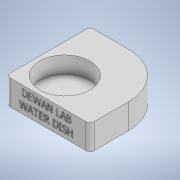
# Autodesk Inventor part: water dish holder_flat
Saved by Autodesk Inventor 2022.2 (Build 262287000, 287)
## iProperties
Created: 2022-03-09
Part Number: water dish holder_flat
Material: Generic
Document SubType Name: Modeling
Designer: dewanlab
Density: 1 g/cm^3
Appearance: Default
Author: dewanlab
Autodesk Inventor part; units mm, degrees
ref_plane "YZ Plane" through (0, 0, 0) normal (1, 0, 0) x (0, 1, 0)
ref_plane "XZ Plane" through (0, 0, 0) normal (0, 1, 0) x (-1, 0, 0)
ref_plane "XY Plane" through (0, 0, 0) normal (0, 0, 1) x (1, 0, 0)
sketch "Sketch1" plane through (0, 0, 0) normal (0, 1, 0) x (-1, 0, 0)
  line L0 (-31.75, -31.75) -> (31.75, -31.75)
  line L1 (31.75, -31.75) -> (31.75, 31.75)
  line L2 (31.75, 31.75) -> (-31.75, 31.75)
  line L3 (-31.75, 31.75) -> (-31.75, -31.75)
  line L4 (-31.75, -31.75) -> (31.75, 31.75) construction
  line L5 (31.75, -31.75) -> (-31.75, 31.75) construction
  point P0 (0, 0)
  dimension "d0" = 63.5
  dimension "d1" = 63.5
  constraints: 12 end point, 2 midpoint, 2 parallel, 1 horizontal, 1 perpendicular
  measures "d0" distance between parallel lines of L0 L2
  measures "d1" distance between parallel lines of L3 L1
extrude "Extrusion1" add sketch "Sketch1" along normal blind 19.05
fillet "Fillet1" radius 34.29 1 edges at (31.75, 9.525, -31.75)
sketch "Sketch2" plane through (0, 19.05, 0) normal (0, 1, 0) x (1, 0, 0)
  circle A0 centre (-9.525, -9.525) radius 19.05
  line L0 (-31.75, 31.75) -> (-31.75, -31.75) projected
  line L1 (-31.75, -31.75) -> (31.75, -31.75) projected
  point P0 (0, 0)
  dimension "d5" = 38.1
  dimension "d6" = 22.225
  dimension "d7" = 22.225
  constraints: 1 centre point
  measures "d5" diameter of A0
  measures "d6" distance from line of A0.centre L0
  measures "d7" distance from line of A0.centre L1
extrude "Extrusion2" cut sketch "Sketch2" against normal blind 12.7
fillet "Fillet2" radius 3.175 3 edges at (31.75, 9.525, 31.75) (-31.75, 9.525, 31.75) (-31.75, 9.525, -31.75)
sketch "Sketch4" plane through (-28.575, 0, 31.75) normal (0, 0, 1) x (1, 0, 0)
  line L0 (0.3237, 17.4668) -> (54.4444, 17.4668) construction
  line L1 (54.4444, 17.4668) -> (54.4444, 2.6465) construction
  line L2 (54.4444, 2.6465) -> (0.3237, 2.6465) construction
  line L3 (0.3237, 2.6465) -> (0.3237, 17.4668) construction
  spline S0 degree 2 poles (13.0168, 14.2799) (13.0168, 13.5841) (12.4528, 12.4644) (11.9794, 12.1515) knots 0 0 0 1 2 2 2
  spline S1 degree 2 poles (11.9794, 12.1515) (11.5924, 11.9087) (10.7979, 11.744) (10.1804, 11.744) knots 0 0 0 1 2 2 2
  line L4 (10.1804, 11.744) -> (9.0113, 11.744)
  line L5 (9.0113, 11.744) -> (9.0113, 16.824)
  line L6 (9.0113, 16.824) -> (10.1681, 16.824)
  spline S2 degree 2 poles (10.1681, 16.824) (10.8844, 16.824) (11.6995, 16.6099) (11.9876, 16.4205) knots 0 0 0 1 2 2 2
  spline S3 degree 2 poles (11.9876, 16.4205) (12.4775, 16.0953) (13.0168, 15.0209) (13.0168, 14.2799) knots 0 0 0 1 2 2 2
  spline S4 degree 2 poles (12.3129, 14.2881) (12.3129, 14.8727) (11.9259, 15.7001) (11.543, 15.9348) knots 0 0 0 1 2 2 2
  spline S5 degree 2 poles (11.543, 15.9348) (11.2713, 16.0953) (10.658, 16.2394) (10.201, 16.2394) knots 0 0 0 1 2 2 2
  line L7 (10.201, 16.2394) -> (9.6864, 16.2394)
  line L8 (9.6864, 16.2394) -> (9.6864, 12.3286)
  line L9 (9.6864, 12.3286) -> (10.201, 12.3286)
  spline S6 degree 2 poles (10.201, 12.3286) (10.6497, 12.3286) (11.329, 12.4726) (11.6048, 12.6661) knots 0 0 0 1 2 2 2
  spline S7 degree 2 poles (11.6048, 12.6661) (11.9588, 12.9049) (12.3129, 13.6953) (12.3129, 14.2881) knots 0 0 0 1 2 2 2
  line L10 (13.7496, 11.744) -> (13.7496, 16.824)
  line L11 (13.7496, 16.824) -> (16.9277, 16.824)
  line L12 (16.9277, 16.824) -> (16.9277, 16.2229)
  line L13 (16.9277, 16.2229) -> (14.4247, 16.2229)
  line L14 (14.4247, 16.2229) -> (14.4247, 14.8315)
  line L15 (14.4247, 14.8315) -> (16.7589, 14.8315)
  line L16 (16.7589, 14.8315) -> (16.7589, 14.2305)
  line L17 (16.7589, 14.2305) -> (14.4247, 14.2305)
  line L18 (14.4247, 14.2305) -> (14.4247, 12.345)
  line L19 (14.4247, 12.345) -> (16.9277, 12.345)
  line L20 (16.9277, 12.345) -> (16.9277, 11.744)
  line L21 (16.9277, 11.744) -> (13.7496, 11.744)
  line L22 (23.3621, 16.824) -> (22.0859, 11.744)
  line L23 (22.0859, 11.744) -> (21.3284, 11.744)
  line L24 (21.3284, 11.744) -> (20.2951, 15.9595)
  line L25 (20.2951, 15.9595) -> (19.2907, 11.744)
  line L26 (19.2907, 11.744) -> (18.5414, 11.744)
  line L27 (18.5414, 11.744) -> (17.2447, 16.824)
  line L28 (17.2447, 16.824) -> (17.9404, 16.824)
  line L29 (17.9404, 16.824) -> (18.9613, 12.6126)
  line L30 (18.9613, 12.6126) -> (19.974, 16.824)
  line L31 (19.974, 16.824) -> (20.6615, 16.824)
  line L32 (20.6615, 16.824) -> (21.6825, 12.5632)
  line L33 (21.6825, 12.5632) -> (22.6993, 16.824)
  line L34 (22.6993, 16.824) -> (23.3621, 16.824)
  line L35 (23.4197, 11.744) -> (25.1322, 16.824)
  line L36 (25.1322, 16.824) -> (25.9638, 16.824)
  line L37 (25.9638, 16.824) -> (27.6764, 11.744)
  line L38 (27.6764, 11.744) -> (26.9642, 11.744)
  line L39 (26.9642, 11.744) -> (26.5031, 13.1642)
  line L40 (26.5031, 13.1642) -> (24.5641, 13.1642)
  line L41 (24.5641, 13.1642) -> (24.1031, 11.744)
  line L42 (24.1031, 11.744) -> (23.4197, 11.744)
  line L43 (26.3179, 13.7406) -> (25.5316, 16.1324)
  line L44 (25.5316, 16.1324) -> (24.7494, 13.7406)
  line L45 (24.7494, 13.7406) -> (26.3179, 13.7406)
  line L46 (31.7931, 11.744) -> (31.0356, 11.744)
  line L47 (31.0356, 11.744) -> (28.7879, 16.1241)
  line L48 (28.7879, 16.1241) -> (28.7879, 11.744)
  line L49 (28.7879, 11.744) -> (28.158, 11.744)
  line L50 (28.158, 11.744) -> (28.158, 16.824)
  line L51 (28.158, 16.824) -> (29.1172, 16.824)
  line L52 (29.1172, 16.824) -> (31.1632, 12.802)
  line L53 (31.1632, 12.802) -> (31.1632, 16.824)
  line L54 (31.1632, 16.824) -> (31.7931, 16.824)
  line L55 (31.7931, 16.824) -> (31.7931, 11.744)
  line L56 (37.9475, 11.744) -> (35.0041, 11.744)
  line L57 (35.0041, 11.744) -> (35.0041, 16.824)
  line L58 (35.0041, 16.824) -> (35.6792, 16.824)
  line L59 (35.6792, 16.824) -> (35.6792, 12.345)
  line L60 (35.6792, 12.345) -> (37.9475, 12.345)
  line L61 (37.9475, 12.345) -> (37.9475, 11.744)
  line L62 (37.931, 11.744) -> (39.6436, 16.824)
  line L63 (39.6436, 16.824) -> (40.4752, 16.824)
  line L64 (40.4752, 16.824) -> (42.1877, 11.744)
  line L65 (42.1877, 11.744) -> (41.4755, 11.744)
  line L66 (41.4755, 11.744) -> (41.0145, 13.1642)
  line L67 (41.0145, 13.1642) -> (39.0755, 13.1642)
  line L68 (39.0755, 13.1642) -> (38.6144, 11.744)
  line L69 (38.6144, 11.744) -> (37.931, 11.744)
  line L70 (40.8292, 13.7406) -> (40.0429, 16.1324)
  line L71 (40.0429, 16.1324) -> (39.2607, 13.7406)
  line L72 (39.2607, 13.7406) -> (40.8292, 13.7406)
  spline S8 degree 2 poles (46.115, 13.3042) (46.115, 12.9255) (45.8269, 12.345) (45.5881, 12.1557) knots 0 0 0 1 2 2 2
  spline S9 degree 2 poles (45.5881, 12.1557) (45.2999, 11.9334) (44.6454, 11.744) (44.1267, 11.744) knots 0 0 0 1 2 2 2
  line L73 (44.1267, 11.744) -> (42.6694, 11.744)
  line L74 (42.6694, 11.744) -> (42.6694, 16.824)
  line L75 (42.6694, 16.824) -> (44.0155, 16.824)
  spline S10 degree 2 poles (44.0155, 16.824) (44.5589, 16.824) (45.1023, 16.754) (45.3493, 16.6182) knots 0 0 0 1 2 2 2
  spline S11 degree 2 poles (45.3493, 16.6182) (45.6252, 16.4741) (45.8763, 16.0006) (45.8763, 15.6795) knots 0 0 0 1 2 2 2
  spline S12 degree 2 poles (45.8763, 15.6795) (45.8763, 15.3214) (45.4975, 14.7533) (45.1641, 14.5927) knots 0 0 0 1 2 2 2
  line L76 (45.1641, 14.5927) -> (45.1641, 14.568)
  spline S13 degree 2 poles (45.1641, 14.568) (45.6169, 14.4445) (46.115, 13.79) (46.115, 13.3042) knots 0 0 0 1 2 2 2
  spline S14 degree 2 poles (45.4111, 13.2754) (45.4111, 13.5636) (45.2464, 13.9341) (44.9994, 14.0658) knots 0 0 0 1 2 2 2
  spline S15 degree 2 poles (44.9994, 14.0658) (44.8389, 14.1481) (44.4601, 14.1975) (44.1102, 14.1975) knots 0 0 0 1 2 2 2
  line L77 (44.1102, 14.1975) -> (43.3445, 14.1975)
  line L78 (43.3445, 14.1975) -> (43.3445, 12.3203)
  line L79 (43.3445, 12.3203) -> (43.892, 12.3203)
  spline S16 degree 2 poles (43.892, 12.3203) (44.3366, 12.3203) (44.8471, 12.4027) (45.0447, 12.5344) knots 0 0 0 1 2 2 2
  spline S17 degree 2 poles (45.0447, 12.5344) (45.2341, 12.6702) (45.4111, 13.0078) (45.4111, 13.2754) knots 0 0 0 1 2 2 2
  spline S18 degree 2 poles (45.1723, 15.5849) (45.1723, 15.766) (45.0488, 16.0377) (44.913, 16.1159) knots 0 0 0 1 2 2 2
  spline S19 degree 2 poles (44.913, 16.1159) (44.7483, 16.2065) (44.349, 16.2476) (43.9908, 16.2476) knots 0 0 0 1 2 2 2
  line L80 (43.9908, 16.2476) -> (43.3445, 16.2476)
  line L81 (43.3445, 16.2476) -> (43.3445, 14.7615)
  line L82 (43.3445, 14.7615) -> (44.1102, 14.7615)
  spline S20 degree 2 poles (44.1102, 14.7615) (44.4272, 14.7615) (44.7277, 14.8274) (44.8883, 14.9303) knots 0 0 0 1 2 2 2
  spline S21 degree 2 poles (44.8883, 14.9303) (45.0447, 15.0291) (45.1723, 15.3461) (45.1723, 15.5849) knots 0 0 0 1 2 2 2
  line L83 (13.1136, 8.4599) -> (11.8374, 3.3799)
  line L84 (11.8374, 3.3799) -> (11.0799, 3.3799)
  line L85 (11.0799, 3.3799) -> (10.0466, 7.5954)
  line L86 (10.0466, 7.5954) -> (9.0421, 3.3799)
  line L87 (9.0421, 3.3799) -> (8.2929, 3.3799)
  line L88 (8.2929, 3.3799) -> (6.9962, 8.4599)
  line L89 (6.9962, 8.4599) -> (7.6919, 8.4599)
  line L90 (7.6919, 8.4599) -> (8.7128, 4.2485)
  line L91 (8.7128, 4.2485) -> (9.7255, 8.4599)
  line L92 (9.7255, 8.4599) -> (10.413, 8.4599)
  line L93 (10.413, 8.4599) -> (11.4339, 4.1991)
  line L94 (11.4339, 4.1991) -> (12.4508, 8.4599)
  line L95 (12.4508, 8.4599) -> (13.1136, 8.4599)
  line L96 (13.1712, 3.3799) -> (14.8837, 8.4599)
  line L97 (14.8837, 8.4599) -> (15.7153, 8.4599)
  line L98 (15.7153, 8.4599) -> (17.4279, 3.3799)
  line L99 (17.4279, 3.3799) -> (16.7157, 3.3799)
  line L100 (16.7157, 3.3799) -> (16.2546, 4.8002)
  line L101 (16.2546, 4.8002) -> (14.3156, 4.8002)
  line L102 (14.3156, 4.8002) -> (13.8546, 3.3799)
  line L103 (13.8546, 3.3799) -> (13.1712, 3.3799)
  line L104 (16.0693, 5.3765) -> (15.2831, 7.7683)
  line L105 (15.2831, 7.7683) -> (14.5009, 5.3765)
  line L106 (14.5009, 5.3765) -> (16.0693, 5.3765)
  line L107 (19.0951, 3.3799) -> (19.0951, 7.8589)
  line L108 (19.0951, 7.8589) -> (17.3908, 7.8589)
  line L109 (17.3908, 7.8589) -> (17.3908, 8.4599)
  line L110 (17.3908, 8.4599) -> (21.4746, 8.4599)
  line L111 (21.4746, 8.4599) -> (21.4746, 7.8589)
  line L112 (21.4746, 7.8589) -> (19.7703, 7.8589)
  line L113 (19.7703, 7.8589) -> (19.7703, 3.3799)
  line L114 (19.7703, 3.3799) -> (19.0951, 3.3799)
  line L115 (21.9892, 3.3799) -> (21.9892, 8.4599)
  line L116 (21.9892, 8.4599) -> (25.1672, 8.4599)
  line L117 (25.1672, 8.4599) -> (25.1672, 7.8589)
  line L118 (25.1672, 7.8589) -> (22.6643, 7.8589)
  line L119 (22.6643, 7.8589) -> (22.6643, 6.4674)
  line L120 (22.6643, 6.4674) -> (24.9985, 6.4674)
  line L121 (24.9985, 6.4674) -> (24.9985, 5.8664)
  line L122 (24.9985, 5.8664) -> (22.6643, 5.8664)
  line L123 (22.6643, 5.8664) -> (22.6643, 3.9809)
  line L124 (22.6643, 3.9809) -> (25.1672, 3.9809)
  line L125 (25.1672, 3.9809) -> (25.1672, 3.3799)
  line L126 (25.1672, 3.3799) -> (21.9892, 3.3799)
  line L127 (29.8397, 3.3799) -> (28.9628, 3.3799)
  line L128 (28.9628, 3.3799) -> (27.3573, 5.4012)
  line L129 (27.3573, 5.4012) -> (26.5834, 5.4012)
  line L130 (26.5834, 5.4012) -> (26.5834, 3.3799)
  line L131 (26.5834, 3.3799) -> (25.9082, 3.3799)
  line L132 (25.9082, 3.3799) -> (25.9082, 8.4599)
  line L133 (25.9082, 8.4599) -> (27.2174, 8.4599)
  spline S22 degree 2 poles (27.2174, 8.4599) (27.6537, 8.4599) (28.2424, 8.3652) (28.51, 8.1923) knots 0 0 0 1 2 2 2
  spline S23 degree 2 poles (28.51, 8.1923) (28.7776, 8.0194) (29.0863, 7.4801) (29.0863, 7.0808) knots 0 0 0 1 2 2 2
  spline S24 degree 2 poles (29.0863, 7.0808) (29.0863, 6.5251) (28.5182, 5.7717) (28.0325, 5.5906) knots 0 0 0 1 2 2 2
  line L134 (28.0325, 5.5906) -> (29.8397, 3.3799)
  spline S25 degree 2 poles (28.3824, 7.0273) (28.3824, 7.2496) (28.2259, 7.5913) (28.0613, 7.7024) knots 0 0 0 1 2 2 2
  spline S26 degree 2 poles (28.0613, 7.7024) (27.9172, 7.7971) (27.5343, 7.8753) (27.2544, 7.8753) knots 0 0 0 1 2 2 2
  line L135 (27.2544, 7.8753) -> (26.5834, 7.8753)
  line L136 (26.5834, 7.8753) -> (26.5834, 5.9652)
  line L137 (26.5834, 5.9652) -> (27.1762, 5.9652)
  spline S27 degree 2 poles (27.1762, 5.9652) (27.4685, 5.9652) (27.9337, 6.0681) (28.0942, 6.2287) knots 0 0 0 1 2 2 2
  spline S28 degree 2 poles (28.0942, 6.2287) (28.2424, 6.3686) (28.3824, 6.7638) (28.3824, 7.0273) knots 0 0 0 1 2 2 2
  spline S29 degree 2 poles (36.4305, 5.9158) (36.4305, 5.2201) (35.8665, 4.1003) (35.3931, 3.7875) knots 0 0 0 1 2 2 2
  spline S30 degree 2 poles (35.3931, 3.7875) (35.0061, 3.5446) (34.2116, 3.3799) (33.5941, 3.3799) knots 0 0 0 1 2 2 2
  line L138 (33.5941, 3.3799) -> (32.425, 3.3799)
  line L139 (32.425, 3.3799) -> (32.425, 8.4599)
  line L140 (32.425, 8.4599) -> (33.5818, 8.4599)
  spline S31 degree 2 poles (33.5818, 8.4599) (34.2981, 8.4599) (35.1132, 8.2458) (35.4013, 8.0565) knots 0 0 0 1 2 2 2
  spline S32 degree 2 poles (35.4013, 8.0565) (35.8912, 7.7312) (36.4305, 6.6568) (36.4305, 5.9158) knots 0 0 0 1 2 2 2
  spline S33 degree 2 poles (35.7266, 5.924) (35.7266, 6.5086) (35.3396, 7.336) (34.9567, 7.5707) knots 0 0 0 1 2 2 2
  spline S34 degree 2 poles (34.9567, 7.5707) (34.685, 7.7312) (34.0716, 7.8753) (33.6147, 7.8753) knots 0 0 0 1 2 2 2
  line L141 (33.6147, 7.8753) -> (33.1001, 7.8753)
  line L142 (33.1001, 7.8753) -> (33.1001, 3.9645)
  line L143 (33.1001, 3.9645) -> (33.6147, 3.9645)
  spline S35 degree 2 poles (33.6147, 3.9645) (34.0634, 3.9645) (34.7427, 4.1086) (35.0185, 4.302) knots 0 0 0 1 2 2 2
  spline S36 degree 2 poles (35.0185, 4.302) (35.3725, 4.5408) (35.7266, 5.3312) (35.7266, 5.924) knots 0 0 0 1 2 2 2
  line L144 (38.9335, 3.3799) -> (36.9657, 3.3799)
  line L145 (36.9657, 3.3799) -> (36.9657, 3.8986)
  line L146 (36.9657, 3.8986) -> (37.612, 3.8986)
  line L147 (37.612, 3.8986) -> (37.612, 7.9412)
  line L148 (37.612, 7.9412) -> (36.9657, 7.9412)
  line L149 (36.9657, 7.9412) -> (36.9657, 8.4599)
  line L150 (36.9657, 8.4599) -> (38.9335, 8.4599)
  line L151 (38.9335, 8.4599) -> (38.9335, 7.9412)
  line L152 (38.9335, 7.9412) -> (38.2871, 7.9412)
  line L153 (38.2871, 7.9412) -> (38.2871, 3.8986)
  line L154 (38.2871, 3.8986) -> (38.9335, 3.8986)
  line L155 (38.9335, 3.8986) -> (38.9335, 3.3799)
  spline S37 degree 2 poles (41.1853, 3.2893) (40.6337, 3.2893) (39.8597, 3.5199) (39.518, 3.6845) knots 0 0 0 1 2 2 2
  line L156 (39.518, 3.6845) -> (39.518, 4.5326)
  line L157 (39.518, 4.5326) -> (39.5674, 4.5326)
  spline S38 degree 2 poles (39.5674, 4.5326) (39.9009, 4.2197) (40.7448, 3.8739) (41.1359, 3.8739) knots 0 0 0 1 2 2 2
  spline S39 degree 2 poles (41.1359, 3.8739) (41.6958, 3.8739) (42.268, 4.3391) (42.268, 4.7219) knots 0 0 0 1 2 2 2
  spline S40 degree 2 poles (42.268, 4.7219) (42.268, 5.0266) (41.9675, 5.4053) (41.6422, 5.5) knots 0 0 0 1 2 2 2
  spline S41 degree 2 poles (41.6422, 5.5) (41.4076, 5.5659) (41.0165, 5.6564) (40.7242, 5.7305) knots 0 0 0 1 2 2 2
  spline S42 degree 2 poles (40.7242, 5.7305) (40.4608, 5.8005) (40.045, 6.0105) (39.8844, 6.1793) knots 0 0 0 1 2 2 2
  spline S43 degree 2 poles (39.8844, 6.1793) (39.728, 6.348) (39.5551, 6.8009) (39.5551, 7.0973) knots 0 0 0 1 2 2 2
  spline S44 degree 2 poles (39.5551, 7.0973) (39.5551, 7.7148) (40.5184, 8.5505) (41.2635, 8.5505) knots 0 0 0 1 2 2 2
  spline S45 degree 2 poles (41.2635, 8.5505) (41.6916, 8.5505) (42.4491, 8.3817) (42.7743, 8.2211) knots 0 0 0 1 2 2 2
  line L158 (42.7743, 8.2211) -> (42.7743, 7.4143)
  line L159 (42.7743, 7.4143) -> (42.7249, 7.4143)
  spline S46 degree 2 poles (42.7249, 7.4143) (42.4821, 7.6366) (41.7246, 7.9659) (41.3088, 7.9659) knots 0 0 0 1 2 2 2
  spline S47 degree 2 poles (41.3088, 7.9659) (40.8395, 7.9659) (40.259, 7.5254) (40.259, 7.1673) knots 0 0 0 1 2 2 2
  spline S48 degree 2 poles (40.259, 7.1673) (40.259, 6.8462) (40.6007, 6.4633) (40.9218, 6.3769) knots 0 0 0 1 2 2 2
  spline S49 degree 2 poles (40.9218, 6.3769) (41.1359, 6.3192) (41.7575, 6.171) (41.9634, 6.1093) knots 0 0 0 1 2 2 2
  spline S50 degree 2 poles (41.9634, 6.1093) (42.4862, 5.9487) (42.9719, 5.3024) (42.9719, 4.829) knots 0 0 0 1 2 2 2
  spline S51 degree 2 poles (42.9719, 4.829) (42.9719, 4.5285) (42.7291, 3.9521) (42.5109, 3.7504) knots 0 0 0 1 2 2 2
  spline S52 degree 2 poles (42.5109, 3.7504) (42.268, 3.5281) (41.6505, 3.2893) (41.1853, 3.2893) knots 0 0 0 1 2 2 2
  line L160 (47.348, 3.3799) -> (46.6728, 3.3799)
  line L161 (46.6728, 3.3799) -> (46.6728, 5.8664)
  line L162 (46.6728, 5.8664) -> (44.3346, 5.8664)
  line L163 (44.3346, 5.8664) -> (44.3346, 3.3799)
  line L164 (44.3346, 3.3799) -> (43.6594, 3.3799)
  line L165 (43.6594, 3.3799) -> (43.6594, 8.4599)
  line L166 (43.6594, 8.4599) -> (44.3346, 8.4599)
  line L167 (44.3346, 8.4599) -> (44.3346, 6.4674)
  line L168 (44.3346, 6.4674) -> (46.6728, 6.4674)
  line L169 (46.6728, 6.4674) -> (46.6728, 8.4599)
  line L170 (46.6728, 8.4599) -> (47.348, 8.4599)
  line L171 (47.348, 8.4599) -> (47.348, 3.3799)
  point P0 (28.575, 0)
  constraints: 2 other
emboss "Emboss2" sketch "Sketch4" operation cut depth 2.54 direction (0, 0, -1)
sketch "Sketch5" plane through (-31.75, 0, -28.575) normal (-1, 0, 0) x (0, 0, 1)
  line L0 (0.3321, 18.3107) -> (57.2618, 18.3107) construction
  line L1 (57.2618, 18.3107) -> (57.2618, 0.5549) construction
  line L2 (57.2618, 0.5549) -> (0.3321, 0.5549) construction
  line L3 (0.3321, 0.5549) -> (0.3321, 18.3107) construction
  spline S0 degree 2 poles (14.4297, 13.656) (14.4297, 12.9603) (13.8657, 11.8406) (13.3923, 11.5277) knots 0 0 0 1 2 2 2
  spline S1 degree 2 poles (13.3923, 11.5277) (13.0053, 11.2848) (12.2108, 11.1201) (11.5933, 11.1201) knots 0 0 0 1 2 2 2
  line L4 (11.5933, 11.1201) -> (10.4241, 11.1201)
  line L5 (10.4241, 11.1201) -> (10.4241, 16.2001)
  line L6 (10.4241, 16.2001) -> (11.5809, 16.2001)
  spline S2 degree 2 poles (11.5809, 16.2001) (12.2972, 16.2001) (13.1123, 15.9861) (13.4005, 15.7967) knots 0 0 0 1 2 2 2
  spline S3 degree 2 poles (13.4005, 15.7967) (13.8904, 15.4715) (14.4297, 14.397) (14.4297, 13.656) knots 0 0 0 1 2 2 2
  spline S4 degree 2 poles (13.7257, 13.6642) (13.7257, 14.2488) (13.3388, 15.0763) (12.9559, 15.3109) knots 0 0 0 1 2 2 2
  spline S5 degree 2 poles (12.9559, 15.3109) (12.6842, 15.4715) (12.0708, 15.6156) (11.6139, 15.6156) knots 0 0 0 1 2 2 2
  line L7 (11.6139, 15.6156) -> (11.0993, 15.6156)
  line L8 (11.0993, 15.6156) -> (11.0993, 11.7047)
  line L9 (11.0993, 11.7047) -> (11.6139, 11.7047)
  spline S6 degree 2 poles (11.6139, 11.7047) (12.0626, 11.7047) (12.7418, 11.8488) (13.0177, 12.0423) knots 0 0 0 1 2 2 2
  spline S7 degree 2 poles (13.0177, 12.0423) (13.3717, 12.281) (13.7257, 13.0714) (13.7257, 13.6642) knots 0 0 0 1 2 2 2
  line L10 (15.1625, 11.1201) -> (15.1625, 16.2001)
  line L11 (15.1625, 16.2001) -> (18.3405, 16.2001)
  line L12 (18.3405, 16.2001) -> (18.3405, 15.5991)
  line L13 (18.3405, 15.5991) -> (15.8376, 15.5991)
  line L14 (15.8376, 15.5991) -> (15.8376, 14.2077)
  line L15 (15.8376, 14.2077) -> (18.1718, 14.2077)
  line L16 (18.1718, 14.2077) -> (18.1718, 13.6066)
  line L17 (18.1718, 13.6066) -> (15.8376, 13.6066)
  line L18 (15.8376, 13.6066) -> (15.8376, 11.7212)
  line L19 (15.8376, 11.7212) -> (18.3405, 11.7212)
  line L20 (18.3405, 11.7212) -> (18.3405, 11.1201)
  line L21 (18.3405, 11.1201) -> (15.1625, 11.1201)
  line L22 (24.7749, 16.2001) -> (23.4988, 11.1201)
  line L23 (23.4988, 11.1201) -> (22.7413, 11.1201)
  line L24 (22.7413, 11.1201) -> (21.708, 15.3356)
  line L25 (21.708, 15.3356) -> (20.7035, 11.1201)
  line L26 (20.7035, 11.1201) -> (19.9543, 11.1201)
  line L27 (19.9543, 11.1201) -> (18.6575, 16.2001)
  line L28 (18.6575, 16.2001) -> (19.3533, 16.2001)
  line L29 (19.3533, 16.2001) -> (20.3742, 11.9888)
  line L30 (20.3742, 11.9888) -> (21.3869, 16.2001)
  line L31 (21.3869, 16.2001) -> (22.0744, 16.2001)
  line L32 (22.0744, 16.2001) -> (23.0953, 11.9394)
  line L33 (23.0953, 11.9394) -> (24.1122, 16.2001)
  line L34 (24.1122, 16.2001) -> (24.7749, 16.2001)
  line L35 (24.8326, 11.1201) -> (26.5451, 16.2001)
  line L36 (26.5451, 16.2001) -> (27.3767, 16.2001)
  line L37 (27.3767, 16.2001) -> (29.0892, 11.1201)
  line L38 (29.0892, 11.1201) -> (28.377, 11.1201)
  line L39 (28.377, 11.1201) -> (27.916, 12.5404)
  line L40 (27.916, 12.5404) -> (25.977, 12.5404)
  line L41 (25.977, 12.5404) -> (25.5159, 11.1201)
  line L42 (25.5159, 11.1201) -> (24.8326, 11.1201)
  line L43 (27.7307, 13.1167) -> (26.9444, 15.5085)
  line L44 (26.9444, 15.5085) -> (26.1623, 13.1167)
  line L45 (26.1623, 13.1167) -> (27.7307, 13.1167)
  line L46 (33.2059, 11.1201) -> (32.4485, 11.1201)
  line L47 (32.4485, 11.1201) -> (30.2007, 15.5003)
  line L48 (30.2007, 15.5003) -> (30.2007, 11.1201)
  line L49 (30.2007, 11.1201) -> (29.5709, 11.1201)
  line L50 (29.5709, 11.1201) -> (29.5709, 16.2001)
  line L51 (29.5709, 16.2001) -> (30.5301, 16.2001)
  line L52 (30.5301, 16.2001) -> (32.5761, 12.1781)
  line L53 (32.5761, 12.1781) -> (32.5761, 16.2001)
  line L54 (32.5761, 16.2001) -> (33.2059, 16.2001)
  line L55 (33.2059, 16.2001) -> (33.2059, 11.1201)
  line L56 (39.3604, 11.1201) -> (36.4169, 11.1201)
  line L57 (36.4169, 11.1201) -> (36.4169, 16.2001)
  line L58 (36.4169, 16.2001) -> (37.0921, 16.2001)
  line L59 (37.0921, 16.2001) -> (37.0921, 11.7212)
  line L60 (37.0921, 11.7212) -> (39.3604, 11.7212)
  line L61 (39.3604, 11.7212) -> (39.3604, 11.1201)
  line L62 (39.3439, 11.1201) -> (41.0565, 16.2001)
  line L63 (41.0565, 16.2001) -> (41.888, 16.2001)
  line L64 (41.888, 16.2001) -> (43.6006, 11.1201)
  line L65 (43.6006, 11.1201) -> (42.8884, 11.1201)
  line L66 (42.8884, 11.1201) -> (42.4273, 12.5404)
  line L67 (42.4273, 12.5404) -> (40.4884, 12.5404)
  line L68 (40.4884, 12.5404) -> (40.0273, 11.1201)
  line L69 (40.0273, 11.1201) -> (39.3439, 11.1201)
  line L70 (42.2421, 13.1167) -> (41.4558, 15.5085)
  line L71 (41.4558, 15.5085) -> (40.6736, 13.1167)
  line L72 (40.6736, 13.1167) -> (42.2421, 13.1167)
  spline S8 degree 2 poles (47.5279, 12.6804) (47.5279, 12.3016) (47.2397, 11.7212) (47.001, 11.5318) knots 0 0 0 1 2 2 2
  spline S9 degree 2 poles (47.001, 11.5318) (46.7128, 11.3095) (46.0582, 11.1201) (45.5395, 11.1201) knots 0 0 0 1 2 2 2
  line L73 (45.5395, 11.1201) -> (44.0822, 11.1201)
  line L74 (44.0822, 11.1201) -> (44.0822, 16.2001)
  line L75 (44.0822, 16.2001) -> (45.4284, 16.2001)
  spline S10 degree 2 poles (45.4284, 16.2001) (45.9718, 16.2001) (46.5152, 16.1301) (46.7622, 15.9943) knots 0 0 0 1 2 2 2
  spline S11 degree 2 poles (46.7622, 15.9943) (47.038, 15.8502) (47.2891, 15.3768) (47.2891, 15.0557) knots 0 0 0 1 2 2 2
  spline S12 degree 2 poles (47.2891, 15.0557) (47.2891, 14.6975) (46.9104, 14.1294) (46.5769, 13.9689) knots 0 0 0 1 2 2 2
  line L76 (46.5769, 13.9689) -> (46.5769, 13.9442)
  spline S13 degree 2 poles (46.5769, 13.9442) (47.0298, 13.8207) (47.5279, 13.1661) (47.5279, 12.6804) knots 0 0 0 1 2 2 2
  spline S14 degree 2 poles (46.824, 12.6515) (46.824, 12.9397) (46.6593, 13.3102) (46.4123, 13.4419) knots 0 0 0 1 2 2 2
  spline S15 degree 2 poles (46.4123, 13.4419) (46.2517, 13.5243) (45.873, 13.5737) (45.5231, 13.5737) knots 0 0 0 1 2 2 2
  line L77 (45.5231, 13.5737) -> (44.7574, 13.5737)
  line L78 (44.7574, 13.5737) -> (44.7574, 11.6965)
  line L79 (44.7574, 11.6965) -> (45.3049, 11.6965)
  spline S16 degree 2 poles (45.3049, 11.6965) (45.7495, 11.6965) (46.26, 11.7788) (46.4576, 11.9105) knots 0 0 0 1 2 2 2
  spline S17 degree 2 poles (46.4576, 11.9105) (46.6469, 12.0464) (46.824, 12.384) (46.824, 12.6515) knots 0 0 0 1 2 2 2
  spline S18 degree 2 poles (46.5852, 14.961) (46.5852, 15.1421) (46.4617, 15.4138) (46.3258, 15.4921) knots 0 0 0 1 2 2 2
  spline S19 degree 2 poles (46.3258, 15.4921) (46.1612, 15.5826) (45.7618, 15.6238) (45.4037, 15.6238) knots 0 0 0 1 2 2 2
  line L80 (45.4037, 15.6238) -> (44.7574, 15.6238)
  line L81 (44.7574, 15.6238) -> (44.7574, 14.1377)
  line L82 (44.7574, 14.1377) -> (45.5231, 14.1377)
  spline S20 degree 2 poles (45.5231, 14.1377) (45.8401, 14.1377) (46.1406, 14.2035) (46.3011, 14.3065) knots 0 0 0 1 2 2 2
  spline S21 degree 2 poles (46.3011, 14.3065) (46.4576, 14.4053) (46.5852, 14.7222) (46.5852, 14.961) knots 0 0 0 1 2 2 2
  line L83 (14.5264, 7.836) -> (13.2503, 2.756)
  line L84 (13.2503, 2.756) -> (12.4928, 2.756)
  line L85 (12.4928, 2.756) -> (11.4595, 6.9715)
  line L86 (11.4595, 6.9715) -> (10.455, 2.756)
  line L87 (10.455, 2.756) -> (9.7058, 2.756)
  line L88 (9.7058, 2.756) -> (8.409, 7.836)
  line L89 (8.409, 7.836) -> (9.1047, 7.836)
  line L90 (9.1047, 7.836) -> (10.1257, 3.6247)
  line L91 (10.1257, 3.6247) -> (11.1384, 7.836)
  line L92 (11.1384, 7.836) -> (11.8259, 7.836)
  line L93 (11.8259, 7.836) -> (12.8468, 3.5753)
  line L94 (12.8468, 3.5753) -> (13.8636, 7.836)
  line L95 (13.8636, 7.836) -> (14.5264, 7.836)
  line L96 (14.5841, 2.756) -> (16.2966, 7.836)
  line L97 (16.2966, 7.836) -> (17.1282, 7.836)
  line L98 (17.1282, 7.836) -> (18.8407, 2.756)
  line L99 (18.8407, 2.756) -> (18.1285, 2.756)
  line L100 (18.1285, 2.756) -> (17.6675, 4.1763)
  line L101 (17.6675, 4.1763) -> (15.7285, 4.1763)
  line L102 (15.7285, 4.1763) -> (15.2674, 2.756)
  line L103 (15.2674, 2.756) -> (14.5841, 2.756)
  line L104 (17.4822, 4.7526) -> (16.6959, 7.1444)
  line L105 (16.6959, 7.1444) -> (15.9138, 4.7526)
  line L106 (15.9138, 4.7526) -> (17.4822, 4.7526)
  line L107 (20.508, 2.756) -> (20.508, 7.235)
  line L108 (20.508, 7.235) -> (18.8037, 7.235)
  line L109 (18.8037, 7.235) -> (18.8037, 7.836)
  line L110 (18.8037, 7.836) -> (22.8874, 7.836)
  line L111 (22.8874, 7.836) -> (22.8874, 7.235)
  line L112 (22.8874, 7.235) -> (21.1831, 7.235)
  line L113 (21.1831, 7.235) -> (21.1831, 2.756)
  line L114 (21.1831, 2.756) -> (20.508, 2.756)
  line L115 (23.402, 2.756) -> (23.402, 7.836)
  line L116 (23.402, 7.836) -> (26.5801, 7.836)
  line L117 (26.5801, 7.836) -> (26.5801, 7.235)
  line L118 (26.5801, 7.235) -> (24.0772, 7.235)
  line L119 (24.0772, 7.235) -> (24.0772, 5.8436)
  line L120 (24.0772, 5.8436) -> (26.4113, 5.8436)
  line L121 (26.4113, 5.8436) -> (26.4113, 5.2425)
  line L122 (26.4113, 5.2425) -> (24.0772, 5.2425)
  line L123 (24.0772, 5.2425) -> (24.0772, 3.3571)
  line L124 (24.0772, 3.3571) -> (26.5801, 3.3571)
  line L125 (26.5801, 3.3571) -> (26.5801, 2.756)
  line L126 (26.5801, 2.756) -> (23.402, 2.756)
  line L127 (31.2526, 2.756) -> (30.3757, 2.756)
  line L128 (30.3757, 2.756) -> (28.7702, 4.7773)
  line L129 (28.7702, 4.7773) -> (27.9963, 4.7773)
  line L130 (27.9963, 4.7773) -> (27.9963, 2.756)
  line L131 (27.9963, 2.756) -> (27.3211, 2.756)
  line L132 (27.3211, 2.756) -> (27.3211, 7.836)
  line L133 (27.3211, 7.836) -> (28.6302, 7.836)
  spline S22 degree 2 poles (28.6302, 7.836) (29.0666, 7.836) (29.6553, 7.7414) (29.9229, 7.5685) knots 0 0 0 1 2 2 2
  spline S23 degree 2 poles (29.9229, 7.5685) (30.1904, 7.3956) (30.4992, 6.8563) (30.4992, 6.457) knots 0 0 0 1 2 2 2
  spline S24 degree 2 poles (30.4992, 6.457) (30.4992, 5.9012) (29.9311, 5.1478) (29.4453, 4.9667) knots 0 0 0 1 2 2 2
  line L134 (29.4453, 4.9667) -> (31.2526, 2.756)
  spline S25 degree 2 poles (29.7952, 6.4034) (29.7952, 6.6257) (29.6388, 6.9674) (29.4741, 7.0786) knots 0 0 0 1 2 2 2
  spline S26 degree 2 poles (29.4741, 7.0786) (29.3301, 7.1733) (28.9472, 7.2515) (28.6673, 7.2515) knots 0 0 0 1 2 2 2
  line L135 (28.6673, 7.2515) -> (27.9963, 7.2515)
  line L136 (27.9963, 7.2515) -> (27.9963, 5.3413)
  line L137 (27.9963, 5.3413) -> (28.5891, 5.3413)
  spline S27 degree 2 poles (28.5891, 5.3413) (28.8813, 5.3413) (29.3465, 5.4442) (29.5071, 5.6048) knots 0 0 0 1 2 2 2
  spline S28 degree 2 poles (29.5071, 5.6048) (29.6553, 5.7448) (29.7952, 6.14) (29.7952, 6.4034) knots 0 0 0 1 2 2 2
  spline S29 degree 2 poles (37.8434, 5.2919) (37.8434, 4.5962) (37.2794, 3.4765) (36.806, 3.1636) knots 0 0 0 1 2 2 2
  spline S30 degree 2 poles (36.806, 3.1636) (36.419, 2.9207) (35.6245, 2.756) (35.007, 2.756) knots 0 0 0 1 2 2 2
  line L138 (35.007, 2.756) -> (33.8378, 2.756)
  line L139 (33.8378, 2.756) -> (33.8378, 7.836)
  line L140 (33.8378, 7.836) -> (34.9946, 7.836)
  spline S31 degree 2 poles (34.9946, 7.836) (35.7109, 7.836) (36.526, 7.622) (36.8142, 7.4326) knots 0 0 0 1 2 2 2
  spline S32 degree 2 poles (36.8142, 7.4326) (37.3041, 7.1074) (37.8434, 6.0329) (37.8434, 5.2919) knots 0 0 0 1 2 2 2
  spline S33 degree 2 poles (37.1394, 5.3002) (37.1394, 5.8847) (36.7525, 6.7122) (36.3696, 6.9468) knots 0 0 0 1 2 2 2
  spline S34 degree 2 poles (36.3696, 6.9468) (36.0979, 7.1074) (35.4845, 7.2515) (35.0276, 7.2515) knots 0 0 0 1 2 2 2
  line L141 (35.0276, 7.2515) -> (34.513, 7.2515)
  line L142 (34.513, 7.2515) -> (34.513, 3.3406)
  line L143 (34.513, 3.3406) -> (35.0276, 3.3406)
  spline S35 degree 2 poles (35.0276, 3.3406) (35.4763, 3.3406) (36.1555, 3.4847) (36.4314, 3.6782) knots 0 0 0 1 2 2 2
  spline S36 degree 2 poles (36.4314, 3.6782) (36.7854, 3.917) (37.1394, 4.7074) (37.1394, 5.3002) knots 0 0 0 1 2 2 2
  line L144 (40.3463, 2.756) -> (38.3786, 2.756)
  line L145 (38.3786, 2.756) -> (38.3786, 3.2747)
  line L146 (38.3786, 3.2747) -> (39.0249, 3.2747)
  line L147 (39.0249, 3.2747) -> (39.0249, 7.3173)
  line L148 (39.0249, 7.3173) -> (38.3786, 7.3173)
  line L149 (38.3786, 7.3173) -> (38.3786, 7.836)
  line L150 (38.3786, 7.836) -> (40.3463, 7.836)
  line L151 (40.3463, 7.836) -> (40.3463, 7.3173)
  line L152 (40.3463, 7.3173) -> (39.7, 7.3173)
  line L153 (39.7, 7.3173) -> (39.7, 3.2747)
  line L154 (39.7, 3.2747) -> (40.3463, 3.2747)
  line L155 (40.3463, 3.2747) -> (40.3463, 2.756)
  spline S37 degree 2 poles (42.5982, 2.6655) (42.0465, 2.6655) (41.2726, 2.896) (40.9309, 3.0607) knots 0 0 0 1 2 2 2
  line L156 (40.9309, 3.0607) -> (40.9309, 3.9087)
  line L157 (40.9309, 3.9087) -> (40.9803, 3.9087)
  spline S38 degree 2 poles (40.9803, 3.9087) (41.3138, 3.5959) (42.1577, 3.25) (42.5488, 3.25) knots 0 0 0 1 2 2 2
  spline S39 degree 2 poles (42.5488, 3.25) (43.1086, 3.25) (43.6809, 3.7152) (43.6809, 4.0981) knots 0 0 0 1 2 2 2
  spline S40 degree 2 poles (43.6809, 4.0981) (43.6809, 4.4027) (43.3803, 4.7815) (43.0551, 4.8761) knots 0 0 0 1 2 2 2
  spline S41 degree 2 poles (43.0551, 4.8761) (42.8205, 4.942) (42.4294, 5.0326) (42.1371, 5.1067) knots 0 0 0 1 2 2 2
  spline S42 degree 2 poles (42.1371, 5.1067) (41.8736, 5.1767) (41.4578, 5.3866) (41.2973, 5.5554) knots 0 0 0 1 2 2 2
  spline S43 degree 2 poles (41.2973, 5.5554) (41.1409, 5.7242) (40.968, 6.177) (40.968, 6.4734) knots 0 0 0 1 2 2 2
  spline S44 degree 2 poles (40.968, 6.4734) (40.968, 7.0909) (41.9313, 7.9266) (42.6764, 7.9266) knots 0 0 0 1 2 2 2
  spline S45 degree 2 poles (42.6764, 7.9266) (43.1045, 7.9266) (43.862, 7.7578) (44.1872, 7.5973) knots 0 0 0 1 2 2 2
  line L158 (44.1872, 7.5973) -> (44.1872, 6.7904)
  line L159 (44.1872, 6.7904) -> (44.1378, 6.7904)
  spline S46 degree 2 poles (44.1378, 6.7904) (43.8949, 7.0127) (43.1375, 7.342) (42.7217, 7.342) knots 0 0 0 1 2 2 2
  spline S47 degree 2 poles (42.7217, 7.342) (42.2524, 7.342) (41.6719, 6.9016) (41.6719, 6.5434) knots 0 0 0 1 2 2 2
  spline S48 degree 2 poles (41.6719, 6.5434) (41.6719, 6.2223) (42.0136, 5.8394) (42.3347, 5.753) knots 0 0 0 1 2 2 2
  spline S49 degree 2 poles (42.3347, 5.753) (42.5488, 5.6954) (43.1704, 5.5472) (43.3762, 5.4854) knots 0 0 0 1 2 2 2
  spline S50 degree 2 poles (43.3762, 5.4854) (43.899, 5.3249) (44.3848, 4.6785) (44.3848, 4.2051) knots 0 0 0 1 2 2 2
  spline S51 degree 2 poles (44.3848, 4.2051) (44.3848, 3.9046) (44.1419, 3.3283) (43.9237, 3.1265) knots 0 0 0 1 2 2 2
  spline S52 degree 2 poles (43.9237, 3.1265) (43.6809, 2.9042) (43.0633, 2.6655) (42.5982, 2.6655) knots 0 0 0 1 2 2 2
  line L160 (48.7609, 2.756) -> (48.0857, 2.756)
  line L161 (48.0857, 2.756) -> (48.0857, 5.2425)
  line L162 (48.0857, 5.2425) -> (45.7474, 5.2425)
  line L163 (45.7474, 5.2425) -> (45.7474, 2.756)
  line L164 (45.7474, 2.756) -> (45.0723, 2.756)
  line L165 (45.0723, 2.756) -> (45.0723, 7.836)
  line L166 (45.0723, 7.836) -> (45.7474, 7.836)
  line L167 (45.7474, 7.836) -> (45.7474, 5.8436)
  line L168 (45.7474, 5.8436) -> (48.0857, 5.8436)
  line L169 (48.0857, 5.8436) -> (48.0857, 7.836)
  line L170 (48.0857, 7.836) -> (48.7609, 7.836)
  line L171 (48.7609, 7.836) -> (48.7609, 2.756)
  point P0 (28.575, 0)
  constraints: 2 other
emboss "Emboss3" sketch "Sketch5" operation cut depth 2.54 direction (1, 0, 0)
body "Solid1"
